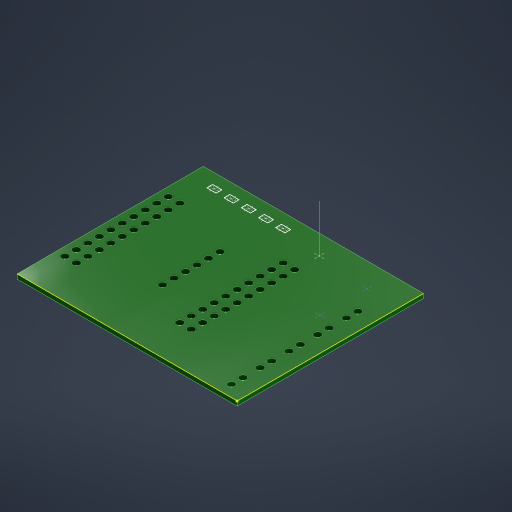
# Autodesk Inventor part: pcb
Saved by Autodesk Inventor 2023 (Build 270158000, 158)
## iProperties
Created: 2022-04-06
Part Number: pcb
Material: Generic
Document SubType Name: Modeling
Designer: Haroon Nawaz
Density: 1 g/cm^3
Appearance: Default
Author: Haroon Nawaz
Autodesk Inventor part; units mm, degrees
ref_plane "YZ Plane" through (0, 0, 0) normal (1, 0, 0) x (0, 1, 0)
ref_plane "XZ Plane" through (0, 0, 0) normal (0, 1, 0) x (-1, 0, 0)
ref_plane "XY Plane" through (0, 0, 0) normal (0, 0, 1) x (1, 0, 0)
sketch "Sketch1" plane through (0, 0, 0) normal (0, 1, 0) x (-1, 0, 0)
  line L0 (0, 0) -> (48.65, 0)
  line L1 (48.65, 0) -> (48.65, -41.19)
  line L2 (48.65, -41.19) -> (0, -41.19)
  line L3 (0, -41.19) -> (0, 0)
  dimension "d0" = 48.65
  dimension "d1" = 41.19
  constraints: 8 end point, 2 parallel, 1 horizontal, 1 perpendicular
  measures "d0" distance of L1.end L2.end
  measures "d1" distance of L0.end L1.end
extrude "Extrusion1" add sketch "Sketch1" along normal blind 1
sketch "Sketch2" plane through (0, 1, 0) normal (0, 1, 0) x (1, 0, 0)
  line L0 (0, 0) -> (-18.8, 0)
  line L1 (-48.65, 0) -> (0, 0) projected
  line L2 (-18.8, 0) -> (-18.8, 8.64)
  line L3 (0, 0) -> (-33.02, 0)
  line L4 (-30.48, 20.32) -> (-30.48, 21.59)
  line L5 (-30.48, 16.51) -> (-30.48, 13.97)
  line L6 (0, 41.19) -> (-48.65, 41.19) projected
  line L7 (0, 0) -> (0, 41.19) projected
  line L8 (-48.65, 41.19) -> (-48.65, 0) projected
  point P0 (-18.8, 11.18)
  point P1 (-18.8, 13.72)
  point P2 (-18.8, 16.26)
  point P3 (-18.8, 18.8)
  point P4 (-18.8, 21.34)
  point P5 (-18.8, 23.88)
  point P6 (-18.8, 26.42)
  point P7 (-18.8, 28.96)
  point P8 (-18.8, 31.5)
  point P9 (-21.34, 8.64)
  point P10 (-21.34, 11.18)
  point P11 (-21.34, 13.72)
  point P12 (-21.34, 16.26)
  point P13 (-21.34, 18.8)
  point P14 (-21.34, 21.34)
  point P15 (-21.34, 23.88)
  point P16 (-21.34, 26.42)
  point P17 (-21.34, 28.96)
  point P18 (-21.34, 31.5)
  point P19 (-30.48, 24.13)
  point P20 (-46.74, 8.64)
  point P21 (-46.74, 8.64)
  point P22 (-46.74, 11.18)
  point P23 (-46.74, 13.72)
  point P24 (-46.74, 16.26)
  point P25 (-46.74, 18.8)
  point P26 (-46.74, 21.34)
  point P27 (-46.74, 23.88)
  point P28 (-46.74, 26.42)
  point P29 (-46.74, 28.96)
  point P30 (-46.74, 31.5)
  point P31 (-44.2, 8.64)
  point P32 (-44.2, 11.18)
  point P33 (-44.2, 13.72)
  point P34 (-44.2, 16.26)
  point P35 (-44.2, 18.8)
  point P36 (-44.2, 21.34)
  point P37 (-44.2, 23.88)
  point P38 (-44.2, 26.42)
  point P39 (-44.2, 28.96)
  point P40 (-44.2, 31.5)
  point P41 (-30.48, 19.05)
  point P42 (-30.48, 19.05)
  point P43 (-30.48, 24.13)
  point P44 (-30.48, 26.67)
  dimension "d4" = 18.8
  dimension "d5" = 8.64
  dimension "d8" = 2.54
  dimension "d11" = 2.54
  dimension "d14" = 33.02
  dimension "d19" = 2.54
  dimension "d26" = 2.54
  dimension "d77" = 41.19
  dimension "d78" = 48.641
  dimension "d89" = 30.48
  constraints: 10 end point, 5 coincident, 3 vertical, 2 point on line, 1 horizontal, 1 perpendicular, 22 other
  measures "d4" distance of L0.start L0.end
  measures "d5" distance of L0.end L2.end
  measures "d8" distance of point (-18.8, 8.64) point (-18.8, 11.18)
  measures "d11" distance of point (-18.8, 8.64) point (-21.34, 8.64)
  measures "d14" distance of L0.start L3.end
  measures "d19" distance of point (-30.48, 21.59) point (-30.48, 24.13)
  measures "d26" distance of point (-30.48, 21.59) point (-30.48, 24.13)
  measures "d77" distance between parallel lines of L0 L6
  measures "d89" distance from line of L7 point (-30.48, 13.97)
hole "Hole1" at (-18.8, 1, -8.64) at (-18.8, 1, -11.18) at (-18.8, 1, -13.72) at (-18.8, 1, -16.26) at (-18.8, 1, -18.8) at (-18.8, 1, -21.34) at (-18.8, 1, -23.88) at (-18.8, 1, -26.42) at (-18.8, 1, -28.96) at (-18.8, 1, -31.5) at (-21.34, 1, -8.64) at (-21.34, 1, -11.18) at (-21.34, 1, -13.72) at (-21.34, 1, -16.26) at (-21.34, 1, -18.8) at (-21.34, 1, -21.34) at (-21.34, 1, -23.88) at (-21.34, 1, -26.42) at (-21.34, 1, -28.96) at (-21.34, 1, -31.5) at (-30.48, 1, -21.59) at (-30.48, 1, -24.13) at (-30.48, 1, -16.51) at (-44.2, 1, -31.5) at (-44.2, 1, -28.96) at (-44.2, 1, -26.42) at (-44.2, 1, -23.88) at (-44.2, 1, -21.34) at (-44.2, 1, -18.8) at (-44.2, 1, -16.26) at (-44.2, 1, -13.72) at (-44.2, 1, -11.18) at (-44.2, 1, -8.64) at (-46.74, 1, -31.5) at (-46.74, 1, -28.96) at (-46.74, 1, -26.42) at (-46.74, 1, -23.88) at (-46.74, 1, -21.34) at (-46.74, 1, -18.8) at (-46.74, 1, -16.26) at (-46.74, 1, -13.72) at (-46.74, 1, -11.18) at (-46.74, 1, -8.64) at (-30.48, 1, -19.05) at (-30.48, 1, -26.67) at (-30.48, 1, -13.97) direction (0, -1, 0) diameter 1.5 end through all
sketch "Sketch3" plane through (0, 1, 0) normal (0, 1, 0) x (1, 0, 0)
  line L0 (-28.956, 38.735) -> (-26.924, 38.735)
  line L1 (-26.924, 38.735) -> (-26.924, 37.465)
  line L2 (-26.924, 37.465) -> (-28.956, 37.465)
  line L3 (-28.956, 37.465) -> (-28.956, 38.735)
  line L4 (-28.956, 38.735) -> (-26.924, 37.465) construction
  line L5 (-26.924, 38.735) -> (-28.956, 37.465) construction
  line L6 (-32.766, 38.735) -> (-30.734, 38.735)
  line L7 (-30.734, 38.735) -> (-30.734, 37.465)
  line L8 (-30.734, 37.465) -> (-32.766, 37.465)
  line L9 (-32.766, 37.465) -> (-32.766, 38.735)
  line L10 (-32.766, 38.735) -> (-30.734, 37.465) construction
  line L11 (-30.734, 38.735) -> (-32.766, 37.465) construction
  line L12 (-36.576, 38.735) -> (-34.544, 38.735)
  line L13 (-34.544, 38.735) -> (-34.544, 37.465)
  line L14 (-34.544, 37.465) -> (-36.576, 37.465)
  line L15 (-36.576, 37.465) -> (-36.576, 38.735)
  line L16 (-36.576, 38.735) -> (-34.544, 37.465) construction
  line L17 (-34.544, 38.735) -> (-36.576, 37.465) construction
  line L18 (-40.386, 38.735) -> (-38.354, 38.735)
  line L19 (-38.354, 38.735) -> (-38.354, 37.465)
  line L20 (-38.354, 37.465) -> (-40.386, 37.465)
  line L21 (-40.386, 37.465) -> (-40.386, 38.735)
  line L22 (-40.386, 38.735) -> (-38.354, 37.465) construction
  line L23 (-38.354, 38.735) -> (-40.386, 37.465) construction
  line L24 (-44.196, 38.735) -> (-42.164, 38.735)
  line L25 (-42.164, 38.735) -> (-42.164, 37.465)
  line L26 (-42.164, 37.465) -> (-44.196, 37.465)
  line L27 (-44.196, 37.465) -> (-44.196, 38.735)
  line L28 (-44.196, 38.735) -> (-42.164, 37.465) construction
  line L29 (-42.164, 38.735) -> (-44.196, 37.465) construction
  line L30 (0, 0) -> (0, 41.19) projected
  line L31 (-48.65, 0) -> (0, 0) projected
  point P0 (-27.94, 38.1)
  point P1 (-31.75, 38.1)
  point P2 (-35.56, 38.1)
  point P3 (-39.37, 38.1)
  point P4 (-43.18, 38.1)
  dimension "d40" = 2.032
  dimension "d41" = 1.27
  dimension "d44" = 3.81
  dimension "d88" = 27.94
  dimension "d90" = 38.1
  constraints: 60 end point, 2 horizontal, 2 midpoint, 2 parallel, 1 collinear, 1 perpendicular, 43 other
  measures "d40" distance of L1.end L2.end
  measures "d41" distance of L0.end L1.end
  measures "d44" distance of L0.start L6.start
  measures "d88" distance from line of L30 point (-27.94, 38.1)
  measures "d90" distance from line of L31 point (-27.94, 38.1)
sketch "Sketch4" plane through (0, 1, 0) normal (0, 1, 0) x (1, 0, 0)
  line L0 (-48.65, 0) -> (0, 0) projected
  line L1 (-3.81, 2.54) -> (-3.81, 5.08)
  line L2 (-3.81, 8.89) -> (-3.81, 11.43)
  line L3 (-3.81, 15.24) -> (-3.81, 17.78)
  line L4 (-3.81, 21.59) -> (-3.81, 24.13)
  line L5 (-3.81, 27.94) -> (-3.81, 30.48)
  point P0 (-3.81, 3.81)
  point P1 (-3.81, 10.16)
  point P2 (-3.81, 16.51)
  point P3 (-3.81, 10.16)
  point P4 (-3.81, 16.51)
  point P5 (-3.81, 16.51)
  point P6 (-3.81, 22.86)
  point P7 (-3.81, 22.86)
  point P8 (-3.81, 22.86)
  point P9 (-3.81, 29.21)
  point P10 (-3.81, 29.21)
  point P11 (-3.81, 29.21)
  dimension "d51" = 3.81
  dimension "d52" = 10.16
  dimension "d53" = 16.51
  dimension "d54" = 1.27
  dimension "d55" = 2.54
  dimension "d58" = 6.35
  dimension "d65" = 6.35
  dimension "d81" = 6.35
  constraints: 10 coincident, 10 end point, 3 collinear, 3 vertical, 26 other
  measures "d51" distance from line of L0 point (-3.81, 3.81)
  measures "d52" distance from line of L0 point (-3.81, 10.16)
  measures "d53" distance from line of L0 point (-3.81, 16.51)
  measures "d54" distance of point (-3.81, 3.81) L1.start
  measures "d55" distance of L1.start L1.end
  measures "d58" distance of L1.start L2.start
  measures "d65" distance of L2.start L3.start
  measures "d81" distance of L3.start L4.start
hole "Hole2" at (-3.81, 1, -2.54) at (-3.81, 1, -5.08) at (-3.81, 1, -8.89) at (-3.81, 1, -11.43) at (-3.81, 1, -17.78) at (-3.81, 1, -15.24) at (-3.81, 1, -21.59) at (-3.81, 1, -24.13) at (-3.81, 1, -27.94) at (-3.81, 1, -30.48) direction (0, -1, 0) diameter 1.5 end through all
sketch "Sketch5" plane through (0, 1, 0) normal (0, 1, 0) x (1, 0, 0)
  line L0 (-48.65, 0) -> (0, 0) projected
  line L1 (0, 0) -> (0, 41.19) projected
  point P0 (-7.239, 25.527)
  point P1 (-18.669, 36.83)
  dimension "d86" = 36.83
  dimension "d87" = 18.669
  measures "d86" distance from line of L0 point (-18.669, 36.83)
  measures "d87" distance from line of L1 point (-18.669, 36.83)
sketch "Sketch6" plane through (0, 1, 0) normal (0, 1, 0) x (1, 0, 0)
  point P0 (0, 0)
  point P1 (-7.112, 35.814)
body "Solid1"
